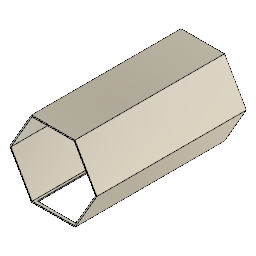
dispenser box hopper v5 (Autodesk Fusion 360 design; units mm, degrees)
Autodesk Fusion 360 part; units mm, degrees
sketch "side" plane through (0, 0, 0) normal (0, 1, 0) x (1, 0, 0)
  line L0 (35, -60.6218) -> (70, 0)
  line L1 (70, 0) -> (35, 60.6218)
  line L2 (35, 60.6218) -> (-35, 60.6218)
  line L3 (-35, 60.6218) -> (-70, 0)
  line L4 (-70, 0) -> (-35, -60.6218)
  line L5 (-35, -60.6218) -> (35, -60.6218)
  dimension "d1" = 70
  constraint horizontal L5
  measures "d1" distance of L0.start L4.end
extrude "Extrude1" add sketch "side" along normal blind 240
sketch "2mm offset cap" plane through (0, 0, 0) normal (0, -1, 0) x (1, 0, 0)
  line L0 (35, 60.6218) -> (-35, 60.6218)
  line L1 (-35, 60.6218) -> (-70, 0)
  line L2 (-70, 0) -> (-35, -60.6218)
  line L3 (-35, -60.6218) -> (35, -60.6218)
  line L4 (35, -60.6218) -> (70, 0)
  line L5 (70, 0) -> (35, 60.6218)
  line L6 (-35, 60.6218) -> (35, 60.6218)
  line L7 (70, 0) -> (35, 60.6218)
  line L8 (70, 0) -> (35, -60.6218)
  line L9 (35, -60.6218) -> (-35, -60.6218)
  line L10 (-35, -60.6218) -> (-70, 0)
  line L11 (-70, 0) -> (-35, 60.6218)
  line L12 (-33.8453, -58.6218) -> (-67.6906, 0)
  line L13 (-67.6906, 0) -> (-33.8453, 58.6218)
  line L14 (-33.8453, 58.6218) -> (33.8453, 58.6218)
  line L15 (67.6906, 0) -> (33.8453, 58.6218)
  line L16 (67.6906, 0) -> (33.8453, -58.6218)
  line L17 (33.8453, -58.6218) -> (-33.8453, -58.6218)
  dimension "d4" = 2
  constraint coincident L0.end L1.start
  constraint coincident L0.start L5.end
  constraint coincident L4.end L5.start
  constraint coincident L3.end L4.start
  constraint coincident L2.end L3.start
  constraint coincident L1.end L2.start
extrude "Extrude2" cut sketch "2mm offset cap" against normal blind 239 contours L12 L13 L14 L15 L16 L17
sketch "opening for tubes" plane through (0, 0, -60.6218) normal (0, 0, -1) x (1, 0, 0)
  line L0 (35, 0) -> (-35, 0)
  line L1 (-35, 0) -> (-35, -240)
  line L2 (-35, -240) -> (35, -240)
  line L3 (35, -240) -> (35, 0)
  line L4 (-35, -240) -> (35, -240)
  line L5 (35, -240) -> (35, 0)
  line L6 (35, 0) -> (-35, 0)
  line L7 (-35, 0) -> (-35, -240)
  line L8 (30, -235) -> (30, -5)
  line L9 (30, -5) -> (-30, -5)
  line L10 (-30, -5) -> (-30, -235)
  line L11 (-30, -235) -> (30, -235)
  dimension "d7" = -5
  constraint horizontal L4
  constraint vertical L5
  constraint horizontal L6
  constraint vertical L7
  constraint coincident L0.start L3.end
  constraint coincident L1.end L2.start
extrude "Extrude4" cut sketch "opening for tubes" against normal blind 2 contours L8 L9 L10 L11
